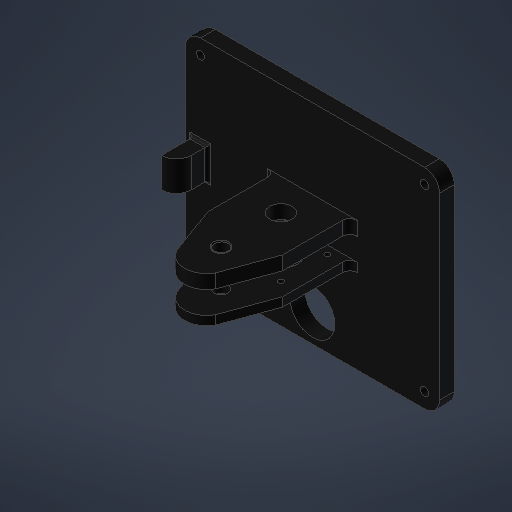
# Autodesk Inventor part: Base
Saved by Autodesk Inventor 2026.2 (Build 302298010, 298A)
## iProperties
Created: 2026-05-30
Part Number: Base
Material: Generic
Document SubType Name: Modeling
Designer: yassi
Density: 1 g/cm^3
Appearance: Smooth - Medium Gray
Author: yassi
## iProperties of the stored document Base_3DPrint.ipt
Created: 2026-06-01
Part Number: Base_3DPrint
Material: Generic
Document SubType Name: Modeling
Designer: yassi
Density: 1 g/cm^3
Appearance: Default
Author: yassi
Autodesk Inventor part; units mm, degrees
ref_plane "YZ Plane" through (0, 0, 0) normal (1, 0, 0) x (0, 1, 0)
ref_plane "XZ Plane" through (0, 0, 0) normal (0, 1, 0) x (-1, 0, 0)
ref_plane "XY Plane" through (0, 0, 0) normal (0, 0, 1) x (1, 0, 0)
sketch "Sketch1" plane through (0, 0, 0) normal (0, 0, 1) x (1, 0, 0)
  line L0 (0, 0) -> (170, 0)
  line L1 (0, 0) -> (0, 140)
  line L2 (0, 140) -> (170, 140)
  line L3 (170, 140) -> (170, 0)
  line L4 (0, 0) -> (10, 0) construction
  dimension "d1" = 170
  dimension "d3" = 140
  constraints: 10 end point, 2 horizontal, 2 perpendicular, 1 coincident, 1 vertical
  measures "d1" distance of L0.start L0.end
  measures "d3" distance of L0.start L1.end
extrude "Extrusion1" add sketch "Sketch1" along normal blind 10
fillet "Fillet1" radius 10 4 edges at (0, 140, 5) (170, 140, 5) (0, 0, 5) (170, 0, 5)
sketch "Sketch2" plane through (0, 0, 10) normal (0, 0, 1) x (1, 0, 0)
  arc A0 (160, 0) -> (170, 10) centre (160, 10) ccw projected
  line L0 (170, 10) -> (170, 130) projected
  arc A1 (170, 130) -> (160, 140) centre (160, 130) ccw projected
  line L1 (160, 140) -> (10, 140) projected
  arc A2 (10, 140) -> (0, 130) centre (10, 130) ccw projected
  line L2 (0, 130) -> (0, 10) projected
  arc A3 (0, 10) -> (10, 0) centre (10, 10) ccw projected
  line L3 (10, 0) -> (160, 0) projected
  line L4 (0, 70) -> (170, 70) construction
  line L5 (0, 130) -> (0, 10) projected
  line L6 (170, 10) -> (170, 130) projected
  line L7 (0, 130) -> (0, 10) projected
  line L8 (60, 77.5) -> (110, 77.5)
  line L9 (60, 86.75) -> (110, 86.75)
  line L10 (110, 62.5) -> (110, 2.5)
  line L11 (110, 2.5) -> (60, 2.5)
  line L12 (60, 2.5) -> (60, 62.5)
  line L13 (60, 62.5) -> (110, 62.5)
  line L14 (60, 56.5) -> (110, 56.5)
  line L15 (60, 77.5) -> (60, 86.75)
  line L16 (110, 77.5) -> (110, 86.75)
  circle A4 centre (10, 130) radius 2.75
  circle A5 centre (10, 10) radius 2.75
  circle A6 centre (160, 130) radius 2.75
  circle A7 centre (160, 10) radius 2.75
  line L17 (5, 80) -> (15, 80)
  line L18 (15, 60) -> (5, 60)
  line L19 (5, 80) -> (5, 60)
  line L20 (15, 80) -> (15, 60)
  line L21 (85, 56.5) -> (85, 11.5)
  circle A8 centre (85, 18.8938) radius 15
  point P0 (0, 0)
  point P1 (5, 70)
  dimension "d18" = 50
  dimension "d75" = 5.5
  dimension "d76" = 5.5
  dimension "d77" = 5.5
  dimension "d83" = 10
  dimension "d84" = 10
  dimension "d85" = 20
  dimension "d92" = 45
  dimension "d93" = 30
  constraints: 30 end point, 6 perpendicular, 5 centre point, 4 coincident, 4 point on line, 3 midpoint, 2 parallel, 1 horizontal, 1 vertical
  measures "d18" distance of L10.end L11.end
  measures "d75" diameter of A4
  measures "d76" diameter of A5
  measures "d77" diameter of A6
  measures "d83" distance of point (5, 70) L17.start
  measures "d84" distance of L17.start L17.end
  measures "d85" distance of L17.end L18.start
  measures "d92" distance of L21.start L21.end
  measures "d93" diameter of A8
extrude "Extrusion2" add sketch "Sketch2" along normal blind 45 contours L10 L14 L12 L13
sketch "Sketch3" plane through (60, 56.5, 10) normal (0, -1, 0) x (1, 0, 0)
  line L0 (50, 0) -> (0, 0) projected
  circle A0 centre (25, 21.15) radius 11.15
  circle A1 centre (9.5, 36.65) radius 1.75
  circle A2 centre (40.5, 36.65) radius 1.75
  circle A3 centre (9.5, 5.65) radius 1.75
  circle A4 centre (40.5, 5.65) radius 1.75
  circle A5 centre (25, 61.15) radius 4.7
  line L1 (0, 0) -> (0, 45) projected
  line L2 (0, 45) -> (11.9707, 77.8892)
  line L3 (0, 45) -> (35, 45) construction
  line L4 (50, 0) -> (50, 45) projected
  line L5 (50, 45) -> (38.0293, 77.8892)
  line L6 (50, 45) -> (85, 45) construction
  line L7 (0, 45) -> (50, 45) projected
  line L8 (0, 45) -> (50, 45)
  arc A6 (38.0293, 77.8892) -> (11.9707, 77.8892) centre (25, 70.7633) ccw
  point P0 (-60, -10)
  dimension "d23" = 22.3
  dimension "d28" = 3.5
  dimension "d29" = 3.5
  dimension "d30" = 3.5
  dimension "d40" = 9.4
  dimension "d42" = 35
  dimension "d43" = 70
  dimension "d44" = 35
  dimension "d45" = 110
  dimension "d80" = 3.5
  constraints: 10 end point, 7 centre point, 2 equal length, 2 horizontal, 2 point on circle, 1 collinear
  measures "d23" diameter of A0
  measures "d28" diameter of A1
  measures "d29" diameter of A2
  measures "d30" diameter of A3
  measures "d40" diameter of A5
  measures "d42" distance of L1.end L2.end
  measures "d43" angle of L3 L2
  measures "d44" distance of L4.end L5.end
  measures "d45" angle of L6 L5
  measures "d80" diameter of A4
extrude "Extrusion3" cut sketch "Sketch3" against normal through all contours A0 | A1 | A2 | A3 | A4
extrude "Extrusion4" add sketch "Sketch2" along normal blind 45 contours L15 L9 L16 L8
sketch "Sketch4" plane through (60, 86.75, 10) normal (0, 1, 0) x (1, 0, 0)
  line L0 (0, 0) -> (50, 0) projected
  line L1 (0, 0) -> (0, -45) projected
  line L2 (50, -45) -> (0, -45) projected
  line L3 (50, 0) -> (50, -45) projected
  circle A0 centre (25, -21.15) radius 11.15 projected
  circle A1 centre (25, -21.15) radius 7.5
  point P0 (-60, 10)
  dimension "d35" = 15
  constraints: 1 centre point, 1 coincident
  measures "d35" diameter of A1
extrude "Extrusion5" cut sketch "Sketch4" against normal through all contours A1
fillet "Fillet2" radius 5 4 edges at (110, 82.125, 10) (60, 82.125, 10) (60, 59.5, 10) (110, 59.5, 10)
extrude "Extrusion6" add sketch "Sketch3" against normal blind 6 contours L7 L2 A6 L5
sketch "Sketch5" plane through (60, 86.75, 55) normal (0, 1, 0) x (1, 0, 0)
  circle A0 centre (25, -16.15) radius 4.7 projected
  circle A1 centre (25, -16.15) radius 4.7
  line L0 (50, 0) -> (38.0293, -32.8892)
  line L1 (50, 0) -> (85, 0) construction
  line L2 (0, 40) -> (0, 0) projected
  line L3 (0, 0) -> (11.9707, -32.8892)
  line L4 (0, 0) -> (35, 0) construction
  arc A2 (11.9707, -32.8892) -> (38.0293, -32.8892) centre (25, -25.7633) ccw
  line L5 (0, 0) -> (50, 0)
  point P0 (-60, 55)
  dimension "d48" = 35
  dimension "d49" = 110
  dimension "d50" = 35
  dimension "d51" = 70
  dimension "d54" = 14.8506
  constraints: 10 end point, 3 horizontal, 2 centre point, 2 equal length, 2 point on circle, 1 coincident
  measures "d48" distance of L0.start L0.end
  measures "d49" angle of L0 L1
  measures "d50" distance of L2.end L3.end
  measures "d51" angle of L3 L4
  measures "d54" radius of A2
extrude "Extrusion7" add sketch "Sketch5" against normal blind 9.25
sketch "Sketch7" plane through (55, 86.75, 10) normal (0, 1, 0) x (1, 0, 0)
  circle A0 centre (30, -61.15) radius 4.7 projected
  circle A1 centre (30, -61.15) radius 5.2
  point P0 (-55, 10)
  dimension "d58" = 10.4
  constraints: 1 centre point, 1 coincident
  measures "d58" diameter of A1
extrude "Extrusion8" add sketch "Sketch7" along normal blind 0.5
fillet "Fillet4" radius 0.75 1 edges at (80.3, 87.25, 71.15)
sketch "Sketch8" plane through (55, 56.5, 10) normal (0, -1, 0) x (1, 0, 0)
  circle A0 centre (30, 61.15) radius 4.7 projected
  circle A1 centre (30, 61.15) radius 5.2
  point P0 (-55, -10)
  dimension "d66" = 10.4
  constraints: 1 centre point, 1 coincident
  measures "d66" diameter of A1
extrude "Extrusion9" add sketch "Sketch8" along normal blind 0.5
fillet "Fillet5" radius 0.75 1 edges at (80.3, 56, 71.15)
fillet "Fillet6" radius 0.75 1 edges at (79.8, 56.5, 71.15)
extrude "Extrusion10" cut sketch "Sketch2" against normal blind 45 contours A4 | A5 | A6 | A7
extrude "Extrusion11" add sketch "Sketch2" along normal blind 21.2 contours L17 L20 L18 L19
fillet "Fillet7" radius 10 1 edges at (15, 70, 31.2)
fillet "Fillet8" radius 2 3 edges at (5, 70, 10) (10, 60, 10) (10, 80, 10)
fillet "Fillet9" radius 2 3 edges at (15, 59, 10) (15, 70, 10) (15, 81, 10)
extrude "Extrusion12" cut sketch "Sketch2" against normal through all contours A8
body "Solid1"
